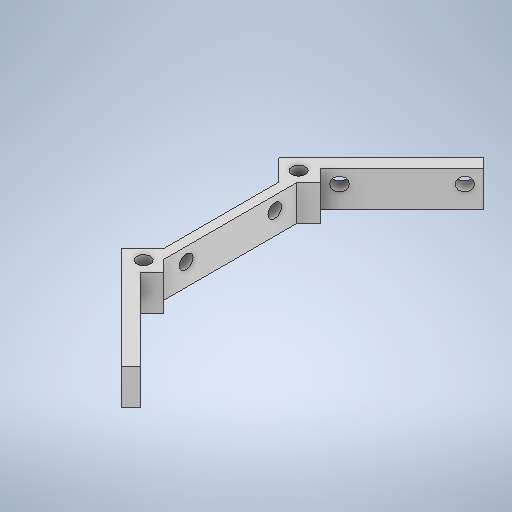
# Autodesk Inventor part: distanceSensorMount
Saved by Autodesk Inventor 2025.1 (Build 291241020, 241B)
## iProperties
Created: 2025-04-15
Part Number: distanceSensorMount
Material: Generic
Document SubType Name: Modeling
Designer: 7008661
Density: 1 g/cm^3
Appearance: Default
Author: 7008661
Autodesk Inventor part; units mm, degrees
ref_plane "YZ Plane" through (0, 0, 0) normal (1, 0, 0) x (0, 1, 0)
ref_plane "XZ Plane" through (0, 0, 0) normal (0, 1, 0) x (-1, 0, 0)
ref_plane "XY Plane" through (0, 0, 0) normal (0, 0, 1) x (1, 0, 0)
sketch "Sketch1" plane through (0, 0, 0) normal (0, 1, 0) x (-1, 0, 0)
  line L0 (0, 22.5) -> (-17.6777, 40.1777)
  line L1 (0, -22.5) -> (-17.6777, -40.1777)
  line L2 (0, 0) -> (0, 13)
  line L3 (0, 13) -> (0, -13)
  line L4 (-17.6777, 40.1777) -> (-19.799, 38.0563)
  line L5 (0, 22.5) -> (-2.1213, 20.3787)
  line L6 (-2.1213, 20.3787) -> (-19.799, 38.0563)
  line L7 (-2.1213, -20.3787) -> (-19.799, -38.0563)
  line L8 (-19.799, -38.0563) -> (-17.6777, -40.1777)
  line L9 (-2.1213, -20.3787) -> (0, -22.5)
  circle A0 centre (0, -17.5) radius 1.525
  circle A1 centre (0, 17.5) radius 1.525
  line L10 (0, -22.5) -> (2, -20.5)
  line L11 (0, -13) -> (2, -15)
  line L12 (0, 22.5) -> (2, 20.5)
  line L13 (0, 13) -> (2, 15)
  line L14 (0, -22.5) -> (-18.3848, -40.8848)
  line L15 (-18.3848, -40.8848) -> (-20.5061, -38.7635)
  line L16 (-20.5061, -38.7635) -> (-19.799, -38.0563)
  line L17 (-19.799, 38.0563) -> (-20.5061, 38.7635)
  line L18 (-20.5061, 38.7635) -> (-18.3848, 40.8848)
  line L19 (-18.3848, 40.8848) -> (-17.6777, 40.1777)
  line L20 (0, -13) -> (-2.1213, -15)
  line L21 (-2.1213, -20.3787) -> (-4.8107, -17.6893)
  line L22 (-2.1213, -20.3787) -> (1.682, -20.3787) construction
  line L23 (-4.8107, -17.6893) -> (-2.1213, -15)
  line L24 (2, -20.5) -> (4.75, -17.75)
  line L25 (4.75, -17.75) -> (2, -15)
  line L26 (0, 13) -> (-2.1213, 15.1213)
  line L27 (-2.1213, 15.1213) -> (-4.75, 17.75)
  line L28 (-4.75, 17.75) -> (-2.1213, 20.3787)
  line L29 (2, 15) -> (4.75, 17.75)
  line L30 (4.75, 17.75) -> (2, 20.5)
  line L31 (-2.1213, -15) -> (-2.1213, 15.1213)
  dimension "d3" = 25
  dimension "d6" = 25
  dimension "d8" = 13
  dimension "d9" = 26
  dimension "d10" = 3
  dimension "d12" = 3.05
  dimension "d13" = 3.05
  dimension "d16" = 26
  dimension "d17" = 135
  constraints: 64 end point, 14 perpendicular, 6 parallel, 2 centre point, 2 point on line, 1 equal length, 1 horizontal
  measures "d3" distance of L0.start L0.end
  measures "d6" distance of L1.start L1.end
  measures "d8" distance of L2.start L2.end
  measures "d9" distance of L2.end L3.end
  measures "d10" distance of L0.end L4.end
  measures "d12" diameter of A0
  measures "d13" diameter of A1
  measures "d16" distance of L1.start L14.end
  measures "d17" angle of L22 L21
extrude "Extrusion2" add sketch "Sketch1" along normal blind 8
sketch "Sketch3" plane through (0, 0, -13) normal (-1, 0, 0) x (0, 0, 1)
  point P0 (13, 0)
sketch "Sketch4" plane through (0, 0, -13) normal (-1, 0, 0) x (0, 0, 1)
  line L0 (13, 0) -> (13, 5)
  line L1 (13, 5) -> (3, 5)
  line L2 (3, 5) -> (23, 5)
  circle A0 centre (3, 5) radius 1.55
  circle A1 centre (23, 5) radius 1.55
  dimension "d20" = 5
  dimension "d21" = 10
  dimension "d22" = 20
  dimension "d23" = 3.1
  dimension "d24" = 3.1
  constraints: 6 end point, 2 centre point, 2 coincident, 1 perpendicular, 1 point on line, 1 vertical
  measures "d20" distance of L0.start L0.end
  measures "d21" distance of L0.end L1.end
  measures "d22" distance of L1.end L2.end
  measures "d23" diameter of A0
  measures "d24" diameter of A1
extrude "Extrusion3" cut sketch "Sketch4" against normal blind 8
sketch "Sketch5" plane through (-4.75, 0, -17.75) normal (-0.7071, 0, -0.7071) x (-0.7071, 0, 0.7071)
  line L0 (-6.7175, 0) -> (-32.7175, 0) projected
  line L1 (-32.7175, 0) -> (-6.7175, 0)
  line L2 (-19.7175, 0) -> (-19.7175, 5)
  line L3 (-19.7175, 5) -> (-29.7175, 5)
  line L4 (-29.7175, 5) -> (-9.7175, 5)
  circle A0 centre (-29.7175, 5) radius 1.55
  circle A1 centre (-9.7175, 5) radius 1.55
  point P0 (9.1924, 0)
  dimension "d27" = 5
  dimension "d28" = 10
  dimension "d29" = 20
  dimension "d30" = 3.1
  dimension "d31" = 3.1
  constraints: 8 end point, 2 centre point, 2 coincident, 1 collinear, 1 midpoint, 1 perpendicular, 1 point on line, 1 vertical
  measures "d27" distance of L2.start L2.end
  measures "d28" distance of L2.end L3.end
  measures "d29" distance of L3.end L4.end
  measures "d30" diameter of A0
  measures "d31" diameter of A1
extrude "Extrusion4" cut sketch "Sketch5" against normal blind 8
sketch "Sketch6" plane through (18.3848, 0, 40.8848) normal (-0.7071, 0, 0.7071) x (0.7071, 0, 0.7071)
  line L0 (-32.7175, 0) -> (0, 0) projected
  line L1 (0, 0) -> (-26, 0)
  line L2 (0, 0) -> (-13, 0)
  line L3 (-13, 0) -> (-13, 5)
  line L4 (-13, 5) -> (-23, 5)
  line L5 (-23, 5) -> (-3, 5)
  circle A0 centre (-23, 5) radius 1.55
  circle A1 centre (-3, 5) radius 1.55
  point P0 (-41.9099, 0)
  dimension "d34" = 26
  dimension "d35" = 13
  dimension "d36" = 5
  dimension "d37" = 10
  dimension "d38" = 20
  dimension "d39" = 3.1
  dimension "d40" = 3.1
  constraints: 10 end point, 2 centre point, 2 coincident, 2 perpendicular, 2 point on line, 1 midpoint
  measures "d34" distance of L0.end L1.end
  measures "d35" distance of L0.end L2.end
  measures "d36" distance of L2.end L3.end
  measures "d37" distance of L3.end L4.end
  measures "d38" distance of L4.end L5.end
  measures "d39" diameter of A0
  measures "d40" diameter of A1
extrude "Extrusion5" cut sketch "Sketch6" against normal blind 8
body "Solid2"
